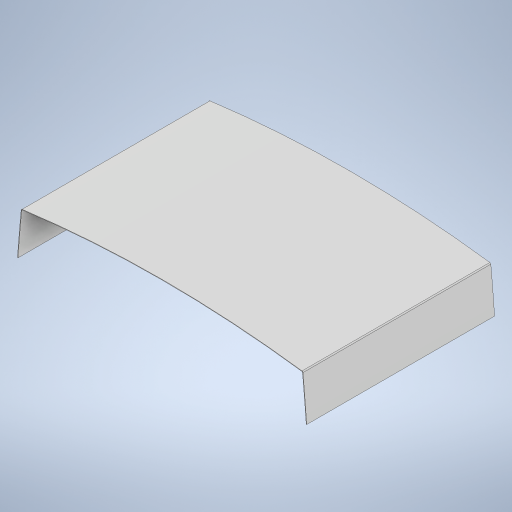
# Autodesk Inventor part: МОО 010 лист спина 1
Saved by Autodesk Inventor 2024.2 (Build 282272000, 272)
## iProperties
Created: 2024-04-18
Part Number: МОО 010 лист спина 1
Material: Stainless Steel AISI 304
Document SubType Name: Sheet Metal
Designer: admin
Density: 8 g/cm^3
Sheet Metal Rule: Default_mm
Sheet Metal Width: 1000,000 mm
Sheet Metal Length: 1966,489 mm
Sheet Metal Area: 1966489,348 mm^2
Appearance: Default
Stock Number: МОО 010 лист спина 1
Flat Pattern Width: 100 cm
Flat Pattern Length: 196.649 cm
Flat Pattern Area: 19664.9 cm^2
Author: admin
Autodesk Inventor part; units mm, degrees
ref_plane "YZ Plane" through (0, 0, 0) normal (1, 0, 0) x (0, 1, 0)
ref_plane "XZ Plane" through (0, 0, 0) normal (0, 1, 0) x (-1, 0, 0)
ref_plane "XY Plane" through (0, 0, 0) normal (0, 0, 1) x (1, 0, 0)
sketch "Sketch1" plane through (0, 0, 0) normal (0, 0, 1) x (1, 0, 0)
  line L0 (-850, 0) -> (850, 0) construction
  line L1 (850, 0) -> (850, -2700) construction
  line L2 (850, -2700) -> (-850, -2700) construction
  line L3 (-850, -2700) -> (-850, 0) construction
  line L4 (-850, 0) -> (850, -2700) construction
  line L5 (850, 0) -> (-850, -2700) construction
  line L6 (-850, -2100) -> (850, -2100) construction
  line L7 (800, -50) -> (-800, -50) construction
  line L8 (-800, -50) -> (-800, -2650) construction
  line L9 (-800, -2650) -> (800, -2650) construction
  line L10 (800, -2650) -> (800, -50) construction
  line L11 (-800, -2100) -> (-110, -2650)
  line L12 (110, -2650) -> (800, -2100)
  line L13 (-750, -100) -> (750, -100) construction
  line L14 (750, -100) -> (750, -2600) construction
  line L15 (750, -2600) -> (-750, -2600) construction
  line L16 (-750, -2600) -> (-750, -100) construction
  arc A0 (750, -100) -> (0, -50) centre (0, -5700) ccw construction
  arc A1 (-750, -100) -> (-750.4642, -104.7339) centre (9627.5218, -1119.9275) ccw construction
  arc A2 (750, -2139.8551) -> (750, -100) centre (-9627.5218, -1119.9275) ccw construction
  line L17 (-110, -2650) -> (110, -2650)
  line L18 (-769.3993, -321.6534) -> (-772.3905, -321.4238) construction
  line L19 (-750, -2139.8551) -> (-752.9856, -2140.1485)
  arc A3 (-772.3905, -321.4238) -> (-752.9856, -2140.1485) centre (9624.5105, -1119.9597) ccw
  line L20 (-750, -100) -> (-747.0144, -100.2934) construction
  line L21 (-767.3573, -334.3434) -> (-770.3488, -334.1173)
  arc A4 (-747.0144, -100.2934) -> (-746.7844, -2142.4182) centre (9630.5107, -1120.1873) ccw construction
  line L22 (-750, -100) -> (-749.6018, -102.9735) construction
  line L23 (750, -100) -> (749.6018, -102.9735) construction
  arc A5 (749.6018, -102.9735) -> (-749.6018, -102.9735) centre (0, -5703.0268) ccw construction
  arc A6 (-744.8882, -102.3445) -> (-747.4784, -105.0263) centre (-744.4927, -105.3183) ccw construction
  arc A7 (-745.2841, -99.3704) -> (-750.4642, -104.7339) centre (-744.4927, -105.318) ccw
  line L24 (0, -50) -> (0, -53.0268) construction
  arc A8 (-745.2841, -99.3704) -> (-750, -100) centre (0, -5700) ccw construction
  arc A9 (-750.4642, -104.7339) -> (-770.3488, -334.1173) centre (9627.5218, -1119.9275) ccw
  arc A10 (-770.3488, -334.1173) -> (-750, -2139.8551) centre (9627.5218, -1119.9275) ccw
  arc A11 (0, -50) -> (-745.2841, -99.3704) centre (0, -5700) ccw
  line L25 (-750, -2139.8551) -> (-751.8699, -2142.201)
  line L26 (-751.8699, -2142.201) -> (-111.8699, -2652.3459)
  line L27 (-111.8699, -2652.3459) -> (-110, -2650)
  line L28 (-110, -2653) -> (111.5183, -2653)
  line L29 (110, -2650) -> (111.5183, -2653)
  line L30 (-110, -2650) -> (-110, -2653)
  point P0 (0, 0)
  point P1 (0, -1350)
  point P2 (0, 0)
  dimension "d18" = 1700
  dimension "d19" = 2700
  dimension "d20" = 2100
  dimension "d22" = 50
  dimension "d23" = 220
  dimension "d24" = 50
  dimension "d29" = 3
  dimension "d32" = 12.5
  dimension "d33" = 235
  dimension "d34" = 3
  dimension "d35" = 6
  measures "d18" distance of L0.start L0.end
  measures "d19" distance of L2.end L0.start
  measures "d20" distance between parallel lines of L0 L6
  measures "d22" distance between parallel lines of L0 L7
  measures "d23" distance of L12.start L11.end
  measures "d24" distance between parallel lines of L7 L13
  measures "d29" distance of L19.start L19.end
  measures "d32" distance of L21.end L18.start
  measures "d33" distance of L13.start L21.end
  measures "d34" radius of A6
  measures "d35" radius of A7
contour flange "Contour Flange2" sketch "Sketch1" thickness 3 bend radius 3 width 1000 along (0, 0, 1) mid plane no both sides no wall seen from (-373.4588, -62.3561, 0) lies toward (0.0660989, -0.9978131, 0) curves A11 A7 A9
bend "Bend2"
corner "Corner2"
mirror "Mirror1" about plane through (0, 0, 0) normal (1, 0, 0) of "Contour Flange2"
equation "\"d18\" = Бак_ширина_общая"
equation "\"d19\" = Бак_высота_общая"
equation "\"d20\" = Бак_высота_до_конуса"
equation "\"d22\" = Бак_высота_ребер_Х"
equation "\"d23\" = Бак_брюхо_ширина_полки"
equation "\"d29\" = Thickness"
equation "\"d32\" = Бак_нахлест_фланца"
equation "\"d33\" = Бак_спина_длина_фланцев"
equation "\"d34\" = Thickness"
equation "\"d35\" = Thickness + BendRadius"
equation "\"d36\" = Thickness"
equation "\"d37\" = BendReliefWidth"
equation "\"d38\" = BendReliefDepth"
equation "\"d39\" = MinimumRemnant"
equation "\"d40\" = TransitionRadius"
equation "\"d42\" = BendRadius"
equation "\"d44\" = CornerReliefSize"
equation "\"d45\" = GapSize"
equation "\"d46\" = JacobiRadiusSize"
equation "\"BendRadius\" = Thickness"
equation "\"BendReliefWidth\" = Thickness"
equation "\"BendReliefDepth\" = 0.5 * Thickness"
equation "\"CornerReliefSize\" = 4 * Thickness"
equation "\"MinimumRemnant\" = 2 * Thickness"
equation "\"TransitionRadius\" = BendRadius"
equation "\"JacobiRadiusSize\" = BendRadius"
equation "\"GapSize\" = Thickness"
equation "\"Бак_ширина_общая\" = 1700"
equation "\"Бак_высота_общая\" = 2700"
equation "\"Бак_высота_до_конуса\" = 2100"
equation "\"Бак_высота_ребер_Х\" = 50"
equation "\"Бак_брюхо_ширина_полки\" = 220"
equation "\"Thickness\" = 3"
equation "\"Бак_нахлест_фланца\" = 12.5"
equation "\"Бак_спина_длина_фланцев\" = 235"
body "Solid3"
